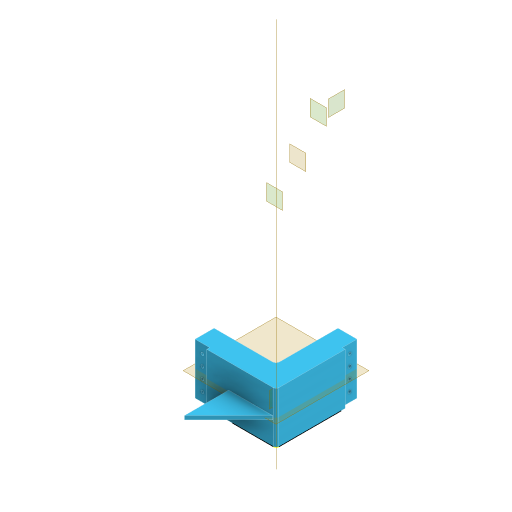
# Autodesk Inventor part: Столбик(задний верх)
Saved by Autodesk Inventor 2023.2 (Build 272271030, 271C)
## iProperties
Created: 2025-04-23
Part Number: Столбик(задний верх)
Material: Типовые
Document SubType Name: Modeling
Designer: Коноваленко
Density: 1 g/cm^3
Appearance: Бирюзовый
Author: Коноваленко
Autodesk Inventor part; units mm, degrees
ref_plane "YZ Plane" through (0, 0, 0) normal (1, 0, 0) x (0, 1, 0)
ref_plane "XZ Plane" through (0, 0, 0) normal (0, 1, 0) x (-1, 0, 0)
ref_plane "XY Plane" through (0, 0, 0) normal (0, 0, 1) x (1, 0, 0)
sketch "Эскиз1" plane through (0, 0, 0) normal (0, 1, 0) x (-1, 0, 0)
  line L0 (-30, -85) -> (-30, 30)
  line L1 (-30, 30) -> (85, 30)
  line L2 (85, 30) -> (85, 0)
  line L3 (85, 0) -> (0, 0)
  line L4 (0, 0) -> (0, -85)
  line L5 (0, -85) -> (-30, -85)
  circle A0 centre (-26, 26) radius 4
  line L6 (85, 26) -> (65, 26)
  line L7 (65, 26) -> (65, 30)
  circle A1 centre (5, -5) radius 5
  line L8 (-30, -85) -> (-26, -85)
  line L9 (-26, -85) -> (-26, -65)
  line L10 (-26, -65) -> (-30, -65)
  line L11 (-30, -65) -> (-30, -85)
  line L12 (0, -85) -> (-4, -85)
  line L13 (0, -65) -> (0, -85)
  line L14 (85, 0) -> (65, 0)
  line L15 (85, 4) -> (85, 0)
  point P0 (-26, 30)
  point P1 (-30, 26)
  point P2 (0, -5)
  point P3 (5, 0)
  dimension "d0" = 115
  dimension "d1" = 115
  dimension "d2" = 30
  dimension "d3" = 30
  dimension "d6" = 4
  dimension "d7" = 20
  dimension "d8" = 10
  dimension "d9" = 4
  dimension "d10" = 20
  dimension "d26" = 8
  constraints: 32 end point, 7 perpendicular, 4 horizontal, 4 point on line, 4 tangent, 2 centre point, 2 parallel, 1 vertical
  measures "d0" distance of L0.end L1.end
  measures "d1" distance of L0.start L0.end
  measures "d2" distance between parallel lines of L1 L3
  measures "d3" distance between parallel lines of L0 L4
  measures "d6" distance between parallel lines of L6 L1
  measures "d7" distance between parallel lines of L2 L7
  measures "d8" diameter of A1
  measures "d9" distance between parallel lines of L0 L9
  measures "d10" distance of L8.end L9.end
  measures "d26" diameter of A0
extrude "Выдавливание1" add sketch "Эскиз1" along normal blind 70 contours L0 A0 L1 L7 L6 L2 L3 L4 L5 L9 L10 | A0 | L4 L3 A1
sketch "Эскиз2" plane through (0, 0, 0) normal (0, -1, 0) x (1, 0, 0)
  line L0 (-5, 0) -> (-85, 0) projected
  line L1 (-30, 0) -> (-30, 30)
  line L2 (-30, 30) -> (26, 30)
  line L3 (30, 26) -> (30, -59)
  line L4 (0, -85) -> (0, -5) projected
  arc A0 (0, -5) -> (-5, 0) centre (-5, -5) ccw projected
  line L5 (0, -85) -> (0, -5) projected
  arc A1 (30, 26) -> (26, 30) centre (26, 26) ccw projected
  line L6 (30, -59) -> (0, -59)
  point P0 (0, 0)
  point P1 (-30, 15)
  point P2 (-65, 0)
  point P3 (0, -65)
  point P4 (0, -59)
  dimension "d134" = 60
  dimension "d135" = 30
  dimension "d136" = 30
  dimension "d137" = 85
  constraints: 8 end point, 4 perpendicular, 2 point on circle, 2 point on line, 1 midpoint
  measures "d134" distance between parallel lines of L3 L1
  measures "d135" distance between parallel lines of L0 L2
  measures "d136" distance between parallel lines of L4 L3
  measures "d137" distance of L3.start L3.end
ref_plane "РабПлоскость2" through (0, 300, -30) normal (0, 0, 1) x (1, 0, 0)
ref_plane "РабПлоскость13" through (23, 363, -35) normal (0, 0, -1) x (-1, 0, 0)
ref_plane "РабПлоскость18" through (25, 57, 23) normal (-1, 0, 0) x (0, 0, 1)
ref_plane "РабПлоскость10" through (-85, 0, -85) normal (0.7071068, 0, -0.7071068) x (0, -1, 0)
ref_plane "РабПлоскость12" through (23, 293, 25) normal (0, 0, -1) x (-1, 0, 0)
ref_plane "РабПлоскость11" through (25, 363, -58) normal (-1, 0, 0) x (0, 0, 1)
shell "Оболочка2" thickness 5 removed faces 3 at (-0.8688, 46.6667, -2.1834) at (0, 23.3333, -58.3333) at (-31.6667, 23.3333, 0)
sketch "Эскиз57" plane through (-60, 5, 25) normal (0, 1, 0) x (1, 0, 0)
  line L0 (85, 85) -> (81, 85) projected
  line L1 (60, 30) -> (60, 105) projected
  line L2 (-20, 4) -> (0, 4) projected
  line L3 (-20, 25) -> (55, 25) projected
  line L4 (-20, 25) -> (-20, 4) projected
  line L5 (81, 105) -> (60, 105) projected
  line L6 (81, 85) -> (81, 105) projected
  line L7 (-2, 4) -> (-2, 25)
  line L8 (81, 87) -> (60, 87)
  point P0 (60, 25)
  dimension "d469" = 18
  dimension "d471" = 18
  constraints: 4 end point, 4 point on line, 2 perpendicular
  measures "d469" distance between parallel lines of L4 L7
  measures "d471" distance between parallel lines of L8 L5
extrude "Выдавливание52" add sketch "Эскиз57" along normal up to surface (60 mm away)
ref_plane "РабПлоскость17" through (-60, 35, 25) normal (0, 1, 0) x (1, 0, 0)
sketch "Эскиз60" plane through (-60, 35, 25) normal (0, 1, 0) x (1, 0, 0)
  line L0 (-2, 25) -> (-2, 4) projected
  line L1 (-2, 4) -> (0, 4) projected
  line L2 (0, 4) -> (0, 0) projected
  line L3 (0, 0) -> (85, 0) projected
  line L4 (85, 0) -> (85, 85) projected
  line L5 (85, 85) -> (81, 85) projected
  line L6 (81, 85) -> (81, 87) projected
  line L7 (81, 87) -> (60, 87) projected
  line L8 (60, 30) -> (60, 87) projected
  arc A0 (55, 25) -> (60, 30) centre (55, 30) ccw projected
  line L9 (-2, 25) -> (55, 25) projected
  point P0 (60, 25)
extrude "Выдавливание53" add sketch "Эскиз60" along normal mid plane 5
sketch "Эскиз61" plane through (25, 5, -60) normal (-1, 0, 0) x (0, 0, 1)
  line L0 (85, 27.5) -> (0, 27.5) projected
  line L1 (55, 0) -> (-2, 0) projected
  line L2 (28.5, 27.5) -> (31.5, 27.5)
  line L3 (31.5, 27.5) -> (31.5, 0)
  line L4 (31.5, 0) -> (28.5, 0)
  line L5 (28.5, 0) -> (28.5, 27.5)
  line L6 (-2, 0) -> (-2, 27.5) projected
  point P0 (60, -5)
  point P1 (28.5, 0)
  dimension "d474" = 3
  dimension "d475" = 30.5
  constraints: 8 end point, 2 parallel, 2 point on line, 1 horizontal, 1 perpendicular
  measures "d474" distance between parallel lines of L3 L5
  measures "d475" distance between parallel lines of L6 L5
extrude "Выдавливание54" add sketch "Эскиз61" along normal blind 10
pattern_linear "Прямоуг.массив15" count 2 spacing 30 along (0, 0, 1) of "Выдавливание54"
mirror "Зеркальное отражение18" about plane through (-85, 0, -85) normal (0.7071068, 0, -0.7071068) of "Выдавливание54", "Прямоуг.массив15"
mirror "Зеркальное отражение19" about plane through (-60, 35, 25) normal (0, 1, 0) of "Выдавливание54", "Прямоуг.массив15", "Зеркальное отражение18"
fillet "Сопряжение29" radius 2 50 edges at (25, 37.5, -45.75) (25, 65, -45.75) (25, 65, -15) (25, 37.5, -15) (25, 37.5, 13.25) (25, 65, 13.25) (13.25, 37.5, 25) (25, 51.25, 25) (13.25, 65, 25) (-15, 65, 25) (-15, 37.5, 25) (-45.75, 37.5, 25) (-45.75, 65, 25) (-62, 37.5, 10.5) (-62, 65, 10.5) (10.5, 37.5, -62) (10.5, 65, -62) (21, 51.25, -60) (25, 51.25, -60) (-60, 51.25, 21) (-60, 51.25, 25) (25, 51.25, -31.5) (20, 37.5, -31.5) (15, 37.5, -30) (20, 65, -31.5) (15, 65, -30) (15, 65, 0) (20, 65, -1.5) (25, 51.25, -1.5) (20, 37.5, -1.5) (15, 37.5, 0) (0, 37.5, 15) (-1.5, 37.5, 20) (-1.5, 51.25, 25) (-1.5, 65, 20) (0, 65, 15) (-30, 65, 15) (-31.5, 65, 20) (-31.5, 51.25, 25) (-31.5, 37.5, 20) (-30, 37.5, 15) (-28.5, 37.5, 20) (-28.5, 51.25, 25) (-28.5, 65, 20) (20, 37.5, -28.5) (25, 51.25, -28.5) (20, 65, -28.5) (25, 32.5, -45.75) (20, 32.5, -31.5) (15, 32.5, -30)
fillet "Сопряжение30" radius 2 32 edges at (24.4142, 31.9142, -32.0858) (25, 17.75, -31.5) (20, 5, -31.5) (15, 5, -30) (20, 5, -28.5) (25, 17.75, -28.5) (18, 32.5, -28.5) (10.5, 32.5, -62) (-62, 32.5, 10.5) (-45.75, 32.5, 25) (-31.5, 5, 20) (-31.5, 18.75, 25) (-31.5, 32.5, 20) (-28.5, 5, 20) (-28.5, 18.75, 25) (-28.5, 32.5, 20) (-30, 32.5, 15) (-15, 32.5, 25) (13.25, 32.5, 25) (0, 32.5, 15) (-1.5, 32.5, 20) (-1.5, 18.75, 25) (-1.5, 5, 20) (0, 5, 15) (20, 5, -1.5) (15, 5, 0) (25, 18.75, 25) (25, 32.5, 13.25) (25, 32.5, -14) (25, 18.75, -1.5) (20, 32.5, -1.5) (15, 32.5, 0)
fillet "Сопряжение31" radius 2 9 edges at (1.5, 64.4142, 24.4142) (1.5, 65, 18) (1.5, 38.0858, 24.4142) (1.5, 37.5, 18) (1.5, 51.25, 25) (1.5, 31.9142, 24.4142) (1.5, 32.5, 18) (1.5, 17.75, 25) (1.5, 5, 19)
fillet "Сопряжение32" radius 2 9 edges at (24.4142, 38.0858, 1.5) (25, 51.25, 1.5) (24.4142, 64.4142, 1.5) (18, 65, 1.5) (18, 37.5, 1.5) (18, 32.5, 1.5) (25, 17.75, 1.5) (24.4142, 31.9142, 1.5) (19, 5, 1.5)
sketch "Эскиз62" plane through (-85, 0, 26) normal (0, 0, 1) x (1, 0, 0)
  line L0 (80, 70) -> (0, 70) projected
  line L1 (10, 70) -> (10, 0) construction
  line L2 (80, 0) -> (0, 0) projected
  line L3 (0, 0) -> (0, 70) projected
  circle A0 centre (10, 57.5) radius 2
  circle A1 centre (10, 42.5) radius 2
  circle A2 centre (10, 27.5) radius 2
  circle A3 centre (10, 12.5) radius 2
  point P0 (85, 0)
  dimension "d485" = 10
  dimension "d486" = 4
  dimension "d487" = 12.5
  dimension "d488" = 15
  dimension "d489" = 15
  dimension "d490" = 15
  constraints: 6 point on line, 4 centre point, 3 equal radius, 2 end point, 1 vertical
  measures "d485" distance between parallel lines of L3 L1
  measures "d486" diameter of A0
  measures "d487" distance from line of L0 A0.centre
  measures "d488" distance of A1.centre A0.centre
  measures "d489" distance of A1.centre A2.centre
  measures "d490" distance of A3.centre A2.centre
extrude "Выдавливание55" cut sketch "Эскиз62" against normal up to surface (26 mm away)
mirror "Зеркальное отражение20" about plane through (-85, 0, -85) normal (0.7071068, 0, -0.7071068) of "Выдавливание55"
sketch "Эскиз63" plane through (-62, 5, 0) normal (0, 1, 0) x (1, 0, 0)
  circle A0 centre (77, 45) radius 3.1
  circle A1 centre (77, 15) radius 3.1
  circle A2 centre (77, -15) radius 3.1
  circle A3 centre (47, -15) radius 3.1
  circle A4 centre (17, -15) radius 3.1
  point P0 (62, 0)
  constraints: 5 centre point, 10 other
extrude "Выдавливание56" cut sketch "Эскиз63" against normal up to surface (5 mm away)
sketch "Эскиз64" plane through (-60, 35, 25) normal (0, 1, 0) x (1, 0, 0)
  line L0 (26, -6) -> (86.6, -6)
  line L1 (86.6, -6) -> (26, -66.6)
  line L2 (26, -66.6) -> (26, -6)
  line L3 (-5, -5) -> (86, -5) projected
  line L4 (-5, -5) -> (86, -5) projected
  arc A0 (86, -5) -> (90, -1) centre (86, -1) ccw projected
  line L5 (86, -5) -> (85.5833, -6)
  line L6 (84.9167, -5) -> (84.5, -6)
  point P0 (60, 25)
  dimension "d495" = 45
  dimension "d496" = 60.6
  dimension "d497" = 1
  dimension "d498" = 0.6
  dimension "d499" = 1
  constraints: 10 end point, 3 point on line, 1 coincident, 1 horizontal, 1 parallel, 1 perpendicular
  measures "d495" angle of L1 L0
  measures "d496" distance of L1.end L0.start
  measures "d497" distance between parallel lines of L3 L0
  measures "d498" horizontal distance of L0.end point (86, -5)
  measures "d499" distance between parallel lines of L5 L6
extrude "Выдавливание57" add sketch "Эскиз64" along normal mid plane 5 contours L0 L1 L2
extrude "Выдавливание58" add sketch "Эскиз64" along normal mid plane 2 contours L6 L3 L5 L0
pattern_linear "Прямоуг.массив16" count 6 spacing 10 along (-1, 0, 0) of "Выдавливание58"
